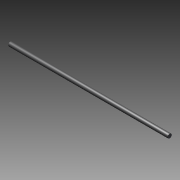
# Autodesk Inventor part: PSFG8-300
Saved by Autodesk Inventor 2011 SP1 (Build 150282100, 282)
## iProperties
Created: 2014-09-26
Part Number: PSFG8-300
Catalog Web Link: www.cadenas.de
Description: SFJ, SFU, SSFJ, SSFU, PSFJ, PSFU, PSSFJ, PSSFU, RSFJ, PSFG, PSSFG-Shafts Solid Type
Vendor: MISUMI
Document SubType Name: Modeling
Designer: psAdmin
Manufacturer: MISUMI
Mass: 15.0736 g
Surface Area: 76.2498 cm^2
Volume: 15.0736 cm^3
Density: 1 g/cm^3
Category: PARTsolutions
Company: MISUMI
Title: PSFG8-300
Author: Cadenas PARTsolutions
Comments: Shafts Solid Type
PSOL_IDENT_0: {\\10.0.0.236\data_v8\23d-libs\misumi\metric\01_linear_shafts\sfj.prj},303 {VTYP=3D},{NB=PSFG8-300},
PSOL_IDENT_1: {LINA=PSFG8-300},{NN=SFJ, SFU, SSFJ, SSFU, PSFJ, PSFU, PSSFJ, PSSFU, RSFJ, PSFG, PSSFG},{DATE=26.08.
PSOL_IDENT_2: 2014 04:38:56},{GEOMDATE=24.07.2014 04:44:00},{VERSION=},{LINEID=50},{LINESUBID=-1},{WBVAR=TS,MAT,ST
PSOL_IDENT_3: ,ALT1,L,ALT3,SC,WSC,X,ALT4,FC,WFC,A,E,ALT5,RC,WRC,Y,ALT6,VC,WVC,F,ALT7,KC,G}  {NB=PSFG8-300},{LINA=P
PSOL_IDENT_4: SFG8-300},{KT=DUMMY},{PN=PSFG8-300},{TYPE=PSFG},{TS=f8},{TSALG= 'g6','g6' , 'h5','h5' , 'f8','f8' },
PSOL_IDENT_5: {MAT=S45C},{MATALG= 'S45C','1045 Carbon Steel' , 'SUS304','304 Stainless Steel' },{HARD=-},{ST=HCP10
PSOL_IDENT_6: },{STALG= 'HCP10','Hard Chrome Plating Plating Hardness: HV750 ~ Plating Thickness: 10 microns or Mo
PSOL_IDENT_7: re' },{D=8},{ALT1=},{L=300.0},{LALG=[20:800/1]},{LMIN=20},{LMAX=800},{LPN=-300},{C=0.5 or Less},{C2=
PSOL_IDENT_8: 0.5},{ALT3=},{ALT3ALG= '','w/o Wrench Flats' , 'SC','with SC (Wrench Flats at One Location)' , 'WSC'
PSOL_IDENT_9: ,'with WSC (Wrench Flats at Two Locations)' },{SC=0},{SCALG=[0]},{SCMAX=292},{WSC=0},{WSCALG=[0]},{W
PSOL_IDENT_10: SCMAX=282},{X=0},{XALG=[0]},{XMAX=282},{WALT3=0},{LL1=0},{LL1ALG=8},{ALT3PN=},{ALT4=},{FC=0},{FCALG=
PSOL_IDENT_11: [0]},{FCMAX=24},{WFC=0},{WFCALG=[0]},{WFCMAX=24},{A=0},{AALG=[0]},{AMAX=0},{E=0},{EALG=[0]},{EMAX=29
PSOL_IDENT_12: 8},{HHALT4=0.0},{ALT4PN=},{ALT5=},{ALT5ALG= '','Not applicable' },{RC=0},{RCALG=[0]},{RCMIN=2},{RCMA
PSOL_IDENT_13: X=300},{WRC=0},{WRCALG=[0]},{WRCMIN=2},{WRCMAX=296},{Y=0},{YALG=[0]},{YMIN=2},{YMAX=298},{BB1=0},{HH
PSOL_IDENT_14: ALT5=0.0},{ALT5PN=},{ALT6=},{ALT6ALG= '','w/o V Groove' , 'VC','with VC (V Groove at One Location)'
PSOL_IDENT_15: , 'WVC','with WVC (V Grooves at Two Locations)' },{VC=0},{VCALG=[0]},{VCMAX=300},{WVC=0},{WVCALG=[0]
PSOL_IDENT_16: },{WVCMIN=2},{WVCMAX=300},{F=0},{FALG=[0]},{FMAX=300},{WALT6=0},{ALT6PN=},{ALT7=},{ALT7ALG= '','Not
PSOL_IDENT_17: applicable' },{KC=0},{KCALG=[0]},{KCMAX1=298},{KCMAX2=300},{G=0},{GALG=[0]},{GMIN=0},{GMAX1=30},{GMA
PSOL_IDENT_18: X2=30},{BB=0},{TT=0.0},{ALT7PN=},{ERRORPN=},{ERRORALT34=OK},{ERRORALT35=OK},{ERRORALT36=OK},{ERRORAL
PSOL_IDENT_19: T37=OK},{ERRORALT45=OK},{ERRORALT46=OK},{ERRORALT47=OK},{ERRORALT56=OK},{ERRORALT57=OK},{ERRORALT67=
PSOL_IDENT_20: OK}
SUPPLIER: MISUMI
ARTICLENO: PSFG8-300
BOMINFO: PSFG8-300
CREATOR: CADENAS GmbH
Autodesk Inventor part; units mm, degrees
ref_plane "YZ Plane" through (0, 0, 0) normal (1, 0, 0) x (0, 1, 0)
ref_plane "XZ Plane" through (0, 0, 0) normal (0, 1, 0) x (-1, 0, 0)
ref_plane "XY Plane" through (0, 0, 0) normal (0, 0, 1) x (1, 0, 0)
sketch "Sketch_3" plane through (0, 0, 0) normal (0, 0, 1) x (1, 0, 0)
  line L0 (300, 0) -> (0, 0)
  line L1 (0, 0) -> (0, 3.5)
  line L2 (0, 3.5) -> (0.5, 4)
  line L3 (0.5, 4) -> (299.5, 4)
  line L4 (299.5, 4) -> (300, 3.5)
  line L5 (300, 3.5) -> (300, 0)
  line L6 (300, 0) -> (0, 0)
  constraints: 14 end point
revolve "Revolution1" add sketch "Sketch_3" angle 360 about axis through (300, 0, 0) along (1, 0, 0)
body "Solid1"
